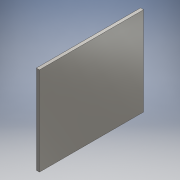
# Autodesk Inventor part: back gusset
Saved by Autodesk Inventor 2016 (Build 200138000, 138)
## iProperties
Created: 2019-03-25
Part Number: back gusset
Material: Stainless Steel, Austenitic
Document SubType Name: Modeling
Designer: benja
Density: 8 g/cm^3
Appearance: Semi-Polished
Mass: 1.632e+06 g
Surface Area: 72440 cm^2
Volume: 204000 cm^3
Author: benja
Autodesk Inventor part; units mm, degrees
ref_plane "YZ Plane" through (0, 0, 0) normal (1, 0, 0) x (0, 1, 0)
ref_plane "XZ Plane" through (0, 0, 0) normal (0, 1, 0) x (-1, 0, 0)
ref_plane "XY Plane" through (0, 0, 0) normal (0, 0, 1) x (1, 0, 0)
sketch "Sketch1" plane through (0, 0, 0) normal (1, 0, 0) x (0, 1, 0)
  line L0 (0, 0) -> (2000, 0)
  line L1 (2000, 0) -> (2000, -1700)
  line L2 (2000, -1700) -> (0, -1700)
  line L3 (0, -1700) -> (0, 0)
  dimension "d0" = 2000
  dimension "d1" = 1700
  constraints: 8 end point, 2 parallel, 1 horizontal, 1 perpendicular
  measures "d0" distance of L1.end L2.end
  measures "d1" distance of L0.end L1.end
extrude "Extrusion1" add sketch "Sketch1" along normal blind 60
body "Solid1"
